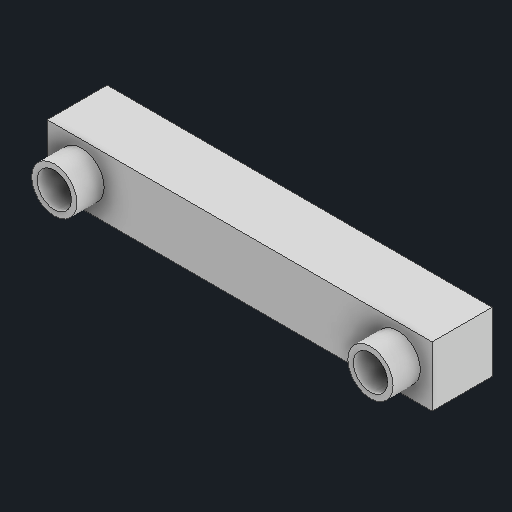
# Autodesk Inventor part: carriage_support
Saved by Autodesk Inventor 2025 (Build 290162010, 162A)
## iProperties
Created: 2024-06-21
Part Number: carriage_support
Material: Generic
Document SubType Name: Modeling
Designer: mihir
Density: 1 g/cm^3
Appearance: Default
Author: mihir
Autodesk Inventor part; units mm, degrees
ref_plane "YZ Plane" through (0, 0, 0) normal (1, 0, 0) x (0, 1, 0)
ref_plane "XZ Plane" through (0, 0, 0) normal (0, 1, 0) x (-1, 0, 0)
ref_plane "XY Plane" through (0, 0, 0) normal (0, 0, 1) x (1, 0, 0)
sketch "Sketch1" plane through (0, 0, 0) normal (0, 1, 0) x (-1, 0, 0)
  line L0 (0, 0) -> (70.6, 0)
  line L1 (70.6, 0) -> (70.6, -11)
  line L2 (70.6, -11) -> (0, -11)
  line L3 (0, -11) -> (0, 0)
  dimension "d0" = 70.6
  dimension "d1" = 11
  constraints: 8 end point, 2 parallel, 1 horizontal, 1 perpendicular
  measures "d0" distance of L1.end L2.end
  measures "d1" distance of L2.end L0.start
extrude "Extrusion1" add sketch "Sketch1" along normal blind 11
sketch "Sketch2" plane through (-70.6, 0, 0) normal (0, 0, 1) x (1, 0, 0)
  circle A0 centre (6.3, 5.5) radius 3.15
  circle A1 centre (64.3, 5.5) radius 3.15
  line L0 (6.3, 5.5) -> (64.3, 5.5) construction
  line L1 (0, 11) -> (70.6, 11) construction
  line L2 (0, 0) -> (0, 11) construction
  circle A2 centre (6.3, 5.5) radius 4.15
  circle A3 centre (64.3, 5.5) radius 4.15
  point P0 (70.6, 0)
  dimension "d4" = 5.5
  dimension "d5" = 58
  dimension "d6" = 6.3
  dimension "d7" = 6.3
  dimension "d8" = 1
  constraints: 4 centre point, 2 coincident, 2 end point, 2 equal radius, 1 horizontal
  measures "d4" distance between parallel lines of L1 L0
  measures "d5" distance of L0.start L0.end
  measures "d6" distance from line of L2 L0.start
  measures "d7" diameter of A0
  measures "d8" radial gap between concentric circles of A2 A0
extrude "Extrusion2" add sketch "Sketch2" along normal blind 5
equation "\"d0\" = carriage_support_length"
equation "\"d1\" = carriage_support_width"
equation "\"d2\" = carriage_support_height"
equation "\"d4\" = 0.5 * carriage_support_height"
equation "\"d5\" = carriage_rod_dist"
equation "\"d6\" = 0.5 * carriage_support_length - 0.5 * carriage_rod_dist"
equation "\"d7\" = carriage_rod_diameter + rod_tolerance"
equation "\"carriage_rod_diameter\" = 6"
equation "\"rod_tolerance\" = 0.3"
equation "\"carriage_support_length\" = 70.6"
equation "\"carriage_support_width\" = 11"
equation "\"carriage_support_height\" = 11"
equation "\"carriage_rod_dist\" = 58"
body "Solid1"
